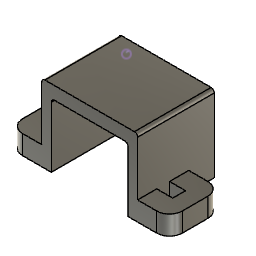
Support_Moteur v2 (Autodesk Fusion 360 design; units mm, degrees)
Autodesk Fusion 360 part; units mm, degrees
sketch "Esquisse1" plane through (0, 0, 0) normal (0, 0, 1) x (1, 0, 0)
  line L0 (0, 0) -> (1.5, 0)
  line L1 (1.5, 0) -> (1.5, 1.2)
  line L2 (1.5, 1.2) -> (0, 1.2)
  line L3 (0, 1.2) -> (0, 0)
  dimension "d1" = 1.5
  dimension "d2" = 1.2
  constraint horizontal L0
  constraint vertical L1
  constraint horizontal L2
  constraint vertical L3
  constraint coincident L0.start L3.end
  measures "d1" distance of L0.start L0.end
  measures "d2" distance of L0.start L2.end
extrude "Extrusion1" add sketch "Esquisse1" along normal blind 1.2
sketch "Esquisse2" plane through (0, 0, 0) normal (0, 0, -1) x (1, 0, 0)
  line L0 (0, 0) -> (0, -1.2)
  line L1 (0, -1.2) -> (1.5, -1.2)
  line L2 (1.5, -1.2) -> (1.5, 0)
  line L3 (1.5, 0) -> (0, 0)
  line L4 (1.35, 0) -> (0.15, 0)
  line L5 (0.15, 0) -> (0.15, -1.2)
  line L6 (0.15, -1.2) -> (1.35, -1.2)
  line L7 (1.35, -1.2) -> (1.35, 0)
  line L8 (0.75, -1.2) -> (0.75, 0)
  dimension "d5" = 1.2
  dimension "d7" = 0.6
  constraint horizontal L4
  constraint vertical L5
  constraint horizontal L6
  constraint vertical L7
  constraint coincident L3 L4.start
  constraint midpoint L1 L8.start
  constraint midpoint L3 L8.end
  measures "d5" distance of L4.start L4.end
  measures "d7" distance of L7 L8
extrude "Extrusion2" cut sketch "Esquisse2" against normal blind 1 contours L1 L3 L4 L5 L6 L8 | L1 L3 L4 L6 L7 L8
sketch "Esquisse3" plane through (1.5, 0, 0) normal (1, 0, 0) x (0, 1, 0)
  line L0 (0, 0) -> (1.2, 0)
  line L1 (1.2, 0) -> (1.2, 1.2)
  line L2 (1.2, 1.2) -> (0, 1.2)
  line L3 (0, 1.2) -> (0, 0)
  line L4 (0, 0) -> (0.8, 0)
  line L5 (0.8, 0) -> (0.8, 0.3)
  line L6 (0.8, 0.3) -> (0, 0.3)
  line L7 (0, 0.3) -> (0, 0)
  dimension "d10" = 0.8
  dimension "d11" = 0.3
  constraint horizontal L4
  constraint vertical L5
  constraint horizontal L6
  constraint vertical L7
  constraint coincident L0.start L3.end
  measures "d10" distance of L0.start L4.end
  measures "d11" distance of L4 L6
extrude "Extrusion3" add sketch "Esquisse3" along normal blind 0.5 contours L0 L3 L4 L5 L6 L7
sketch "Esquisse4" plane through (0, 0, 0.3) normal (0, 0, 1) x (-1, 0, 0)
  line L0 (-1.5, -0.8) -> (-1.5, 0)
  line L1 (-1.5, 0) -> (-2, 0)
  line L2 (-2, 0) -> (-2, -0.8)
  line L3 (-2, -0.8) -> (-1.5, -0.8)
  line L4 (-1.5, -0.5) -> (-1.75, -0.5)
  line L5 (-1.75, -0.5) -> (-1.75, -0.3)
  line L6 (-1.75, -0.3) -> (-1.5, -0.3)
  line L7 (-1.5, -0.3) -> (-1.5, -0.5)
  line L8 (-1.5, -0.4) -> (-2, -0.4)
  dimension "d14" = 0.4
  dimension "d15" = 0.1
  dimension "d16" = 0.2
  dimension "d27" = 0.25
  constraint horizontal L4
  constraint vertical L5
  constraint horizontal L6
  constraint vertical L7
  constraint coincident L0 L4.start
  constraint coincident L0 L8.start
  constraint coincident L2 L8.end
  constraint perpendicular L2 L8
  measures "d14" distance of L3 L8
  measures "d15" distance of L6 L8
  measures "d16" distance of L4 L6
  measures "d27" distance of L5.end L6.end
extrude "Extrusion4" cut sketch "Esquisse4" against normal blind 0.5 contours L0 L4 L5 L7 L8 | L0 L5 L6 L7 L8
sketch "Esquisse5" plane through (0, 0, 0.3) normal (0, 0, 1) x (-1, 0, 0)
  line L0 (-1.75, -0.3) -> (-1.5, -0.3)
  line L1 (-1.5, -0.3) -> (-1.5, 0)
  line L2 (-1.5, 0) -> (-2, 0)
  line L3 (-2, 0) -> (-2, -0.8)
  line L4 (-2, -0.8) -> (-1.5, -0.8)
  line L5 (-1.5, -0.8) -> (-1.5, -0.5)
  line L6 (-1.5, -0.5) -> (-1.75, -0.5)
  line L7 (-1.75, -0.5) -> (-1.75, -0.3)
sketch "Esquisse6" plane through (0, 0, 0) normal (-1, 0, 0) x (0, -1, 0)
  line L0 (-1.2, 0) -> (0, 0)
  line L1 (0, 0) -> (0, 1.2)
  line L2 (0, 1.2) -> (-1.2, 1.2)
  line L3 (-1.2, 1.2) -> (-1.2, 0)
  line L4 (0, 0) -> (-0.8, 0)
  line L5 (-0.8, 0) -> (-0.8, 0.3)
  line L6 (-0.8, 0.3) -> (0, 0.3)
  line L7 (0, 0.3) -> (0, 0)
  dimension "d19" = 0.8
  dimension "d20" = 0.3
  constraint horizontal L4
  constraint vertical L5
  constraint horizontal L6
  constraint vertical L7
  constraint coincident L0.end L1.start
  measures "d19" distance of L0.end L4.end
  measures "d20" distance of L0.end L6.end
extrude "Extrusion5" add sketch "Esquisse6" along normal blind 0.5 contours L0 L1 L4 L5 L6 L7
sketch "Esquisse7" plane through (0, 0, 0.3) normal (0, 0, 1) x (-1, 0, 0)
  line L0 (0, 0) -> (0, -0.8)
  line L1 (0, -0.8) -> (0.5, -0.8)
  line L2 (0.5, -0.8) -> (0.5, 0)
  line L3 (0.5, 0) -> (0, 0)
  line L4 (0, -0.4) -> (0.5, -0.4)
  line L5 (0, -0.3) -> (0.25, -0.3)
  line L6 (0.25, -0.3) -> (0.25, -0.5)
  line L7 (0.25, -0.5) -> (0, -0.5)
  line L8 (0, -0.5) -> (0, -0.3)
  dimension "d23" = 0.25
  dimension "d24" = 0.2
  constraint midpoint L0 L4.start
  constraint midpoint L2 L4.end
  constraint horizontal L5
  constraint vertical L6
  constraint horizontal L7
  constraint vertical L8
  constraint coincident L0 L5.start
  measures "d23" distance of L5.start L5.end
  measures "d24" distance of L5.start L7.end
extrude "Extrusion6" cut sketch "Esquisse7" against normal blind 0.6 contours L0 L4 L5 L6 L8 | L0 L4 L6 L7 L8
fillet "Congé1" radius 0.2 4 edges at (2, 0, 0.15) (2, 0.8, 0.15) (-0.5, 0, 0.15) (-0.5, 0.8, 0.15)
fillet "Congé2" radius 0.05 2 edges at (1.5, 0.6, 1.2) (0, 0.6, 1.2)
fillet "Congé3" radius 0.05 2 edges at (1.35, 0.6, 1) (0.15, 0.6, 1)
scale "Echelle1" factor 10 about (0.05, 1.2, 1.2) bodies 1
